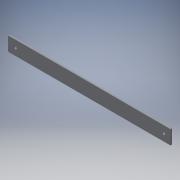
# Autodesk Inventor part: supports
Saved by Autodesk Inventor 2018 (Build 220112000, 112)
## iProperties
Created: 2019-01-20
Part Number: supports
Material: Generic
Document SubType Name: Modeling
Designer: Burni
Density: 1 g/cm^3
Appearance: Default
Mass: 17.9196 g
Surface Area: 157.406 cm^2
Volume: 17.9196 cm^3
Author: Burni
Autodesk Inventor part; units mm, degrees
ref_plane "YZ Plane" through (0, 0, 0) normal (1, 0, 0) x (0, 1, 0)
ref_plane "XZ Plane" through (0, 0, 0) normal (0, 1, 0) x (-1, 0, 0)
ref_plane "XY Plane" through (0, 0, 0) normal (0, 0, 1) x (1, 0, 0)
sketch "Sketch1" plane through (0, 0, 0) normal (0, 0, 1) x (1, 0, 0)
  line L0 (0, 0) -> (279.4, 0)
  line L1 (279.4, 0) -> (279.4, 25.4)
  line L2 (279.4, 25.4) -> (0, 25.4)
  line L3 (0, 25.4) -> (0, 0)
  dimension "d2" = 279.4
  dimension "d3" = 25.4
  constraints: 8 end point, 2 parallel, 1 horizontal, 1 perpendicular
  measures "d2" distance of L1.end L2.end
  measures "d3" distance of L0.end L1.end
extrude "Extrusion1" add sketch "Sketch1" along normal blind 2.54
sketch "Sketch2" plane through (0, 0, 0) normal (0, 0, -1) x (-1, 0, 0)
  circle A0 centre (-12.7, 12.7) radius 2.5797
  line L0 (0, 25.4) -> (0, 0) projected
  line L1 (0, 0) -> (-279.4, 0) projected
  dimension "d6" = 5.1594
  dimension "d7" = 12.7
  dimension "d8" = 12.7
  constraints: 1 centre point
  measures "d6" diameter of A0
  measures "d7" distance from line of L0 A0.centre
  measures "d8" distance from line of L1 A0.centre
extrude "Extrusion2" cut sketch "Sketch2" against normal blind 25.4
sketch "Sketch3" plane through (0, 0, 2.54) normal (0, 0, 1) x (1, 0, 0)
  circle A0 centre (266.7, 12.7) radius 2.5797
  line L0 (279.4, 0) -> (279.4, 25.4) projected
  line L1 (0, 0) -> (279.4, 0) projected
  dimension "d11" = 5.1594
  dimension "d12" = 12.7
  dimension "d13" = 12.7
  constraints: 1 centre point
  measures "d11" diameter of A0
  measures "d12" distance from line of L0 A0.centre
  measures "d13" distance from line of L1 A0.centre
extrude "Extrusion3" cut sketch "Sketch3" against normal blind 25.4
body "Solid1"
